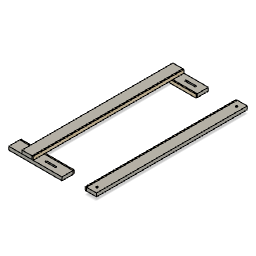
dado-jig (Autodesk Fusion 360 design; units mm, degrees)
Autodesk Fusion 360 part; units mm, degrees
note: some values were not read from the file. Set by a fixed rule: which sketch regions a step uses.
sketch "perpendicular guides" plane through (0, 0, 0) normal (0, 1, 0) x (1, 0, 0)
  line L0 (0, 0) -> (304.8, 0)
  line L1 (304.8, 0) -> (304.8, 63.5)
  line L2 (304.8, 63.5) -> (0, 63.5)
  line L3 (0, 63.5) -> (0, 0)
  line L4 (76.2, 863.6) -> (279.4, 863.6)
  line L5 (279.4, 863.6) -> (279.4, 800.1)
  line L6 (279.4, 800.1) -> (76.2, 800.1)
  line L7 (76.2, 800.1) -> (76.2, 863.6)
  circle A0 centre (181.7687, 831.85) radius 3.9688
  circle A1 centre (237.3312, 831.85) radius 3.9688
  line L8 (76.2, 831.85) -> (279.4, 831.85) construction
  line L9 (181.7687, 835.8187) -> (237.3312, 835.8187)
  line L10 (181.7705, 827.8813) -> (237.333, 827.8813)
  line L11 (241.3, 863.6) -> (241.3, 800.1) construction
  line L12 (177.8, 863.6) -> (177.8, 800.1) construction
  line L13 (181.7687, 831.85) -> (237.3312, 831.85) construction
  line L14 (181.7687, 831.85) -> (237.3312, 831.85) construction
  circle A2 centre (181.7687, 31.75) radius 3.9688
  circle A3 centre (237.3313, 31.75) radius 3.9688
  line L15 (237.3312, 863.6) -> (237.3313, 0) construction
  line L16 (0, 31.75) -> (304.8, 31.75) construction
  line L17 (181.7687, 863.6) -> (181.7687, 0) construction
  line L18 (181.7687, 27.7812) -> (237.3313, 27.7812)
  line L19 (181.7687, 35.7187) -> (237.3313, 35.7187)
  line L20 (241.3, 63.5) -> (241.3, 0) construction
  line L21 (304.8, 63.5) -> (0, 63.5)
  line L22 (0, 63.5) -> (0, 69.85)
  line L23 (0, 69.85) -> (304.8, 69.85)
  line L24 (304.8, 69.85) -> (304.8, 63.5)
  line L25 (279.4, 800.1) -> (76.2, 800.1)
  line L26 (76.2, 800.1) -> (76.2, 793.75)
  line L27 (76.2, 793.75) -> (279.4, 793.75)
  line L28 (279.4, 793.75) -> (279.4, 800.1)
  dimension "d1" = 304.8
  dimension "d2" = 63.5
  dimension "d3" = 152.4
  dimension "d4" = 203.2
  dimension "d7" = 7.9375
  dimension "d8" = 38.1
  dimension "d9" = 101.6
  dimension "d10" = 63.5
  dimension "d11" = 6.35
  dimension "d12" = 6.35
  dimension "d17" = 863.6
  constraint horizontal L0
  constraint vertical L1
  constraint horizontal L2
  constraint vertical L3
  constraint coincident L0.start L3.end
  constraint horizontal L4
  constraint vertical L5
  constraint horizontal L6
  constraint vertical L7
  constraint equal L3 L7
  constraint equal A0 A1
  constraint coincident L7 L8.start
  constraint coincident L5 L8.end
  constraint perpendicular L5 L8
  constraint midpoint L5 L8.end
  constraint coincident A1.centre L8
  constraint coincident A0.centre L8
  constraint coincident A0 L9.start
  constraint coincident A1 L9.end
  constraint tangent A1 L9
  constraint coincident A0 L10.start
  constraint coincident A1 L10.end
  constraint coincident L4 L11.start
  constraint coincident L6 L11.end
  constraint perpendicular L6 L11
  constraint tangent A1 L11
  constraint coincident L4 L12.start
  constraint coincident L6 L12.end
  constraint perpendicular L6 L12
  constraint tangent A0 L12
  constraint parallel L8 L9
  constraint parallel L8 L10
  constraint coincident A0.centre L13.start
  constraint coincident A1.centre L13.end
  constraint equal L10 L13
  constraint equal L9 L10
  constraint equal A1 A3
  constraint equal A1 A2
  constraint coincident L4 L15.start
  constraint coincident L0 L15.end
  constraint perpendicular L0 L15
  constraint coincident A1.centre L15
  constraint coincident L3 L16.start
  constraint coincident L1 L16.end
  constraint perpendicular L1 L16
  constraint midpoint L1 L16.end
  constraint coincident A3.centre L16
  constraint coincident A3.centre L15
  constraint coincident L4 L17.start
  constraint coincident L0 L17.end
  constraint perpendicular L0 L17
  constraint coincident A0.centre L17
  constraint coincident A2.centre L17
  constraint coincident A2.centre L16
  constraint coincident L17 L18.start
  constraint coincident L15 L18.end
  constraint perpendicular L15 L18
  constraint coincident L17 L19.start
  constraint coincident L15 L19.end
  constraint perpendicular L15 L19
  constraint tangent A2 L19
  constraint tangent A2 L18
  constraint coincident L2 L20.start
  constraint coincident L0 L20.end
  constraint perpendicular L0 L20
  constraint tangent A3 L20
  constraint horizontal L21
  constraint vertical L22
  constraint horizontal L23
  constraint vertical L24
  constraint horizontal L25
  constraint vertical L26
  constraint horizontal L27
  constraint vertical L28
  constraint collinear L7 L26
  constraint collinear L3 L22
  measures "d1" distance of L0.start L0.end
  measures "d2" distance of L0.start L2.end
  measures "d4" distance of L4.start L4.end
  measures "d7" diameter of A0
  measures "d8" distance of L5 L11
  measures "d9" distance of L5 L12
  measures "d10" distance of L1 L20
  measures "d11" distance of L2 L23
  measures "d12" distance of L6.end L26.end
  measures "d17" distance of L0 L4
extrude "Extrude1" add sketch "perpendicular guides" along normal blind 19.05 contours L4 L5 L6 L7 L25 makes body 1 in component "top perpendicular"
sketch "long stretch" plane through (0, 19.05, 0) normal (0, 1, 0) x (-1, 0, 0)
  line L0 (-279.4, -800.1) -> (-279.4, -863.6)
  line L1 (-279.4, -863.6) -> (-76.2, -863.6)
  line L2 (-76.2, -863.6) -> (-76.2, -800.1)
  line L3 (-279.4, -863.6) -> (-76.2, -863.6)
  line L4 (0, 0) -> (-304.8, 0)
  line L5 (-76.2, -863.6) -> (-177.8, -863.6) construction
  line L6 (-177.8, 0) -> (-76.2, 0) construction
  line L7 (-76.2, -863.6) -> (-133.35, -863.6)
  line L8 (-133.35, -863.6) -> (-133.35, 0)
  line L9 (-133.35, 0) -> (-76.2, 0)
  line L10 (-76.2, 0) -> (-76.2, -863.6)
  line L11 (-133.35, 0) -> (-139.7, 0)
  line L12 (-139.7, 0) -> (-139.7, -863.6)
  line L13 (-139.7, -863.6) -> (-133.35, -863.6)
  line L14 (-133.35, -863.6) -> (-133.35, 0)
  line L15 (-445.0629, -863.6) -> (-502.2129, -863.6)
  line L16 (-502.2129, -863.6) -> (-502.2129, 0)
  line L17 (-502.2129, 0) -> (-445.0629, 0)
  line L18 (-445.0629, 0) -> (-445.0629, -863.6)
  line L19 (-445.0629, -863.6) -> (-438.7129, -863.6)
  line L20 (-438.7129, -863.6) -> (-438.7129, 0)
  line L21 (-438.7129, 0) -> (-445.0629, 0)
  line L22 (-445.0629, 0) -> (-445.0629, -863.6)
  circle A0 centre (-473.6379, -831.85) radius 3.9687
  circle A1 centre (-473.6379, -31.75) radius 3.9687
  circle A2 centre (-237.3313, -31.75) radius 3.9687 construction
  circle A3 centre (-237.3312, -831.85) radius 3.9687 construction
  line L23 (-502.2129, -831.85) -> (-200.66, -831.85) construction
  line L24 (-502.2129, -31.75) -> (-213.36, -31.75) construction
  line L25 (-445.0629, -31.75) -> (-502.2129, -31.75) construction
  line L26 (-445.0629, -831.85) -> (-502.2129, -831.85) construction
  circle A4 centre (-473.6379, -833.4375) radius 3.9687
  circle A5 centre (-473.6379, -830.2625) radius 3.9687
  line L27 (-445.0629, -833.4375) -> (-502.2129, -833.4375) construction
  line L28 (-502.2129, -837.4062) -> (-439.42, -837.4062) construction
  line L29 (-445.0629, -826.2937) -> (-502.2129, -826.2937) construction
  line L30 (-502.2129, -830.2625) -> (-445.0629, -830.2625) construction
  line L31 (-473.6379, -833.4375) -> (-473.6379, -830.2625) construction
  circle A6 centre (-473.6379, -33.3375) radius 3.9687
  circle A7 centre (-473.6379, -30.1625) radius 3.9687
  line L32 (-502.2129, -30.1625) -> (-445.0629, -30.1625) construction
  line L33 (-445.0629, -33.3375) -> (-502.2129, -33.3375) construction
  line L34 (-480.1105, -33.3375) -> (-480.1105, -31.75) construction
  line L35 (-482.3649, -31.75) -> (-482.3649, -30.1625) construction
  line L36 (-445.0629, -37.3063) -> (-502.2129, -37.3063) construction
  line L37 (-445.0629, -26.1938) -> (-502.2129, -26.1938) construction
  line L38 (-469.6691, -33.3375) -> (-469.6691, -30.1625)
  line L39 (-477.6066, -33.3375) -> (-477.6066, -30.1625)
  line L40 (-469.6691, -833.4375) -> (-469.6691, -830.2625)
  line L41 (-477.6066, -833.4375) -> (-477.6066, -830.2625)
  arc A8 (-181.7687, -835.8188) -> (-181.7705, -827.8813) centre (-181.7687, -831.85) ccw
  line L42 (-181.7687, -835.8188) -> (-237.3312, -835.8188)
  arc A9 (-237.333, -827.8813) -> (-237.3312, -835.8188) centre (-237.3313, -831.85) ccw
  line L43 (-237.333, -827.8813) -> (-181.7705, -827.8813)
  line L44 (-279.4, -800.1) -> (-279.4, -863.6)
  line L45 (-279.4, -863.6) -> (-76.2, -863.6)
  line L46 (-76.2, -863.6) -> (-76.2, -800.1)
  line L47 (-76.2, -800.1) -> (-279.4, -800.1)
  dimension "d15" = 57.15
  dimension "d16" = 6.35
  dimension "d24" = 57.15
  dimension "d25" = 557.2513
  dimension "d26" = 6.35
  dimension "d35" = 11.1125
  dimension "d36" = 11.1125
  constraint horizontal L5
  constraint horizontal L6
  constraint coincident L4 L6.start
  constraint coincident L1.end L2.start
  constraint horizontal L7
  constraint vertical L8
  constraint horizontal L9
  constraint vertical L10
  constraint coincident L6 L8.end
  constraint horizontal L11
  constraint vertical L12
  constraint horizontal L13
  constraint vertical L14
  constraint coincident L3 L12.end
  constraint horizontal L15
  constraint vertical L16
  constraint horizontal L17
  constraint vertical L18
  constraint equal L10 L18
  constraint collinear L1 L15
  constraint horizontal L19
  constraint vertical L20
  constraint horizontal L21
  constraint vertical L22
  constraint collinear L17 L21
  constraint equal A1 A2
  constraint equal A0 A3
  constraint coincident L16 L23.start
  constraint perpendicular L16 L23
  constraint coincident A3.centre L23
  constraint coincident A0.centre L23
  constraint coincident L16 L24.start
  constraint perpendicular L16 L24
  constraint coincident A2.centre L24
  constraint coincident A1.centre L24
  constraint coincident L24 L25.start
  constraint coincident L22 L25.start
  constraint midpoint A1.centre L25
  constraint coincident L23 L26.start
  constraint coincident L22 L26.start
  constraint midpoint A0.centre L26
  constraint equal A4 A5
  constraint equal A0 A5
  constraint collinear A0.centre A4.centre A5.centre
  constraint coincident L22 L27.start
  constraint coincident L16 L27.end
  constraint perpendicular L16 L27
  constraint midpoint A4.centre L27
  constraint coincident L16 L28.start
  constraint perpendicular L16 L28
  constraint coincident L22 L29.start
  constraint coincident L16 L29.end
  constraint perpendicular L16 L29
  constraint tangent A4 L28
  constraint tangent A5 L29
  constraint coincident L16 L30.start
  constraint coincident L22 L30.end
  constraint perpendicular L22 L30
  constraint coincident A5.centre L30
  constraint coincident A4.centre L31.start
  constraint coincident A5.centre L31.end
  constraint perpendicular L30 L31
  constraint midpoint A0.centre L31
  constraint coincident L16 L32.start
  constraint coincident L22 L32.end
  constraint perpendicular L22 L32
  constraint coincident L18 L33.start
  constraint coincident L16 L33.end
  constraint perpendicular L16 L33
  constraint midpoint A6.centre L33
  constraint midpoint A7.centre L32
  constraint equal A1 A7
  constraint equal A1 A6
  constraint coincident L33 L34.start
  constraint coincident L24 L34.end
  constraint perpendicular L24 L34
  constraint coincident L25 L35.start
  constraint coincident L32 L35.end
  constraint perpendicular L32 L35
  constraint equal L34 L35
  constraint coincident L22 L36.start
  constraint coincident L16 L36.end
  constraint perpendicular L16 L36
  constraint coincident L18 L37.start
  constraint coincident L16 L37.end
  constraint perpendicular L16 L37
  constraint tangent A7 L37
  constraint tangent A6 L36
  constraint coincident L33 L38.start
  constraint coincident L32 L38.end
  constraint perpendicular L32 L38
  constraint coincident L33 L39.start
  constraint coincident L32 L39.end
  constraint perpendicular L32 L39
  constraint tangent A6 L38
  constraint tangent A6 L39
  constraint coincident L27 L40.start
  constraint coincident L30 L40.end
  constraint perpendicular L30 L40
  constraint tangent A4 L40
  constraint coincident L27 L41.start
  constraint coincident L30 L41.end
  constraint perpendicular L30 L41
  constraint tangent A4 L41
  measures "d15" distance of L8 L10
  measures "d16" distance of L8 L12
  measures "d24" distance of L15.start L15.end
  measures "d26" distance of L18 L20
  measures "d35" distance of L28 L29
  measures "d36" distance of L36 L37
extrude "Extrude1'" add sketch "perpendicular guides" along normal blind 19.05 separate body contours L0 L1 L2 L3 L21 makes body 2 in component "bottom perpendicular"
extrude "Extrude1''" add sketch "perpendicular guides" along normal blind 19.05 separate body contours L2 L21 L22 L23 L24 makes body 3 in component "bottom liner"
extrude "Extrude2" add sketch "perpendicular guides" along normal blind 19.05 separate body contours L6 L25 L26 L27 L28 makes body 4 in component "top liner"
extrude "Extrude1'''" add sketch "long stretch" along normal blind 19.05 separate body contours L1 L2 L3 L7 L8 L10 L14 L45 L46 L47 | L4 L8 L9 L10 L14 L47 makes body 5 in component "long stretch"
extrude "Extrude1''''" add sketch "long stretch" along normal blind 19.05 separate body contours L1 L3 L8 L12 L13 L14 L45 L47 | L4 L8 L11 L12 L14 L47 makes body 6 in component "long stretch runner"
extrude "Extrude1'''''" add sketch "long stretch" along normal blind 19.05 separate body contours L15 L16 L17 L18 L22 | A0 A4 L40 | A0 A5 L40 | A0 A5 | A0 A4 | A0 A5 L41 | A0 A4 L41 | A1 A6 L38 | A1 A7 L38 | A1 A7 | A1 A6 | A1 A7 L39 | A1 A6 L39 makes body 7 in component "long stretch slider"
extrude "Extrude1''''''" add sketch "long stretch" along normal blind 19.05 separate body contours L18 L19 L20 L21 L22 makes body 8 in component "long stretch slider runner"
sketch "Sketch3" plane through (0, 38.1, 0) normal (0, 1, 0) x (-1, 0, 0)
  circle A0 centre (-473.6379, -31.75) radius 3.9688
  circle A1 centre (-473.6379, -831.85) radius 3.9688
  line L0 (-445.0629, 0) -> (-502.2129, 0)
  line L1 (-502.2129, 0) -> (-502.2129, -863.6)
  line L2 (-502.2129, -863.6) -> (-445.0629, -863.6)
  line L3 (-445.0629, -863.6) -> (-445.0629, 0)
  circle A2 centre (-473.6379, -833.4375) radius 3.9687
  circle A3 centre (-473.6379, -830.2625) radius 3.9687
  line L4 (-469.6691, -833.4375) -> (-469.6691, -830.2625)
  line L5 (-477.6066, -833.4375) -> (-477.6066, -830.2625)
  circle A4 centre (-473.6379, -33.3375) radius 3.9687
  line L6 (-469.6691, -33.3375) -> (-469.6691, -30.1625)
  line L7 (-477.6066, -33.3375) -> (-477.6066, -30.1625)
  circle A5 centre (-473.6379, -30.1625) radius 3.9687
extrude "Extrude2'" cut sketch "Sketch3" against normal blind 1.5875 contours A0 A4 A5 | A0 A4 L6 | A0 L6 A5 | A0 A4 A5 | A0 A5 | A0 A4 | A0 A4 A5 | A0 A4 A5 | A0 L7 A5 | A4 A5 | A0 A4 L7 | A1 A2 A3 | A1 A2 L4 | A1 A3 L4 | A1 A2 A3 | A1 A3 | A1 A2 | A1 A2 A3 | A1 A2 A3 | A1 A3 L5 | A2 A3 | A1 A2 L5 bodies 7 in component "long stretch slider"
component "top perpendicular" placed x (1, 0, 0) y (0, 1, 0) z (0, 0, 1) at (0, 0, 0)
component "bottom perpendicular" placed x (1, 0, 0) y (0, 1, 0) z (0, 0, 1) at (0, 0, 0)
component "bottom liner" placed x (1, 0, 0) y (0, 1, 0) z (0, 0, 1) at (0, 0, 0)
component "long stretch slider" placed x (1, 0, 0) y (0, 1, 0) z (0, 0, 1) at (0, 0, 0)
component "long stretch runner" placed x (1, 0, 0) y (0, 1, 0) z (0, 0, 1) at (0, 0, 0)
component "long stretch" placed x (1, 0, 0) y (0, 1, 0) z (0, 0, 1) at (0, 0, 0)
component "long stretch slider runner" placed x (1, 0, 0) y (0, 1, 0) z (0, 0, 1) at (0, 0, 0)
component "top liner" placed x (1, 0, 0) y (0, 1, 0) z (0, 0, 1) at (0, 0, 0)
equation "d7 = ( 5 / 16 ) * 1 in"
equation "d35 = ( 7 / 16 ) * 1 in"
equation "d36 = ( 7 / 16 ) * 1 in"
equation "plywood_width = 0.75 in"
equation "d42 = plywood_width"
equation "d44 = plywood_width"
equation "d48 = plywood_width"
equation "d50 = plywood_width"
equation "d52 = plywood_width"
equation "d54 = plywood_width"
equation "d56 = plywood_width"
equation "d58 = plywood_width"
equation "d60 = ( -1 / 16 ) * 1 in"
